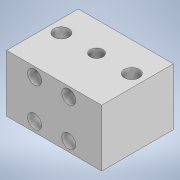
# Autodesk Inventor part: NewSink
Saved by Autodesk Inventor 2020 (Build 240168000, 168)
## iProperties
Created: 2019-09-11
Part Number: NewSink
Material: Generic
Document SubType Name: Modeling
Designer: colman
Density: 1 g/cm^3
Appearance: Default
Author: colman
Autodesk Inventor part; units mm, degrees
ref_plane "YZ Plane" through (0, 0, 0) normal (1, 0, 0) x (0, 1, 0)
ref_plane "XZ Plane" through (0, 0, 0) normal (0, 1, 0) x (-1, 0, 0)
ref_plane "XY Plane" through (0, 0, 0) normal (0, 0, 1) x (1, 0, 0)
sketch "Sketch1" plane through (0, 0, 0) normal (0, 0, 1) x (1, 0, 0)
  line L0 (8.25, 4.95) -> (-8.25, 4.95)
  line L1 (-8.25, 4.95) -> (-8.25, -4.95)
  line L2 (-8.25, -4.95) -> (8.25, -4.95)
  line L3 (8.25, -4.95) -> (8.25, 4.95)
  point P0 (0, 0)
  dimension "d19" = 9.9
  constraints: 8 end point, 2 parallel, 1 horizontal, 1 perpendicular
  measures "d19" distance of L1.end L0.end
extrude "Box" add sketch "Sketch1" along normal mid plane 12.446
sketch "Sketch3" plane through (0, 0, -6.223) normal (0, 0, -1) x (-1, 0, 0)
  line L0 (-5.08, 0) -> (5.08, 0) construction
  line L1 (-4.75, 0) -> (4.75, 0) construction
  line L2 (-2.972, -1.778) -> (2.972, -1.778)
  line L3 (2.972, 1.778) -> (-2.972, 1.778)
  arc A0 (-2.972, 1.778) -> (-2.972, -1.778) centre (-2.972, 0) ccw
  arc A1 (2.972, -1.778) -> (2.972, 1.778) centre (2.972, 0) ccw
  point P0 (0, 0)
  point P1 (0, 0)
  point P2 (0, 0)
  dimension "d31" = 9.5
  constraints: 12 end point, 6 point on circle, 4 point on line, 4 tangent, 2 centre point, 2 midpoint, 1 parallel
  measures "d31" distance of L1.start L1.end
extrude "Slot" cut sketch "Sketch3" against normal blind 10.16
sketch "Sketch4" plane through (0, 0, -6.223) normal (0, 0, -1) x (-1, 0, 0)
  circle A0 centre (-2.5426, 3.364) radius 1.2
  line L0 (-2.972, 1.778) -> (2.972, 1.778) projected
  line L1 (8.25, 4.95) -> (-8.25, 4.95) projected
  point P0 (0, 0)
  dimension "d32" = 2.4
  dimension "d33" = 3.172
  dimension "d34" = 1.586
  constraints: 1 centre point
  measures "d32" diameter of A0
  measures "d33" distance between parallel lines of L0 L1
  measures "d34" distance from line of A0.centre L1
extrude "MountingHole" cut sketch "Sketch4" against normal blind 12.5
pattern_linear "Mounting Holes" count 2 spacing 5.92 along (-1, 0, 0) count 2 spacing 6.648 along (0, -1, 0) of "MountingHole"
sketch "Sketch6" plane through (-8.25, 4.95, 6.223) normal (0, 1, 0) x (1, 0, 0)
  circle A0 centre (8.25, 7.366) radius 1.105
  point P0 (8.25, 6.223)
  dimension "d20" = 2.21
  constraints: 1 centre point
  measures "d20" diameter of A0
extrude "CentralSMAHole" cut sketch "Sketch6" against normal blind 10
sketch "Sketch8" plane through (-8.25, 4.95, 6.223) normal (0, 1, 0) x (1, 0, 0)
  circle A0 centre (14.36, 7.366) radius 1.295
  point P0 (8.25, 6.223)
  dimension "d23" = 2.59
  constraints: 1 centre point
  measures "d23" diameter of A0
extrude "SMAMounting" cut sketch "Sketch8" against normal blind 10
pattern_linear "SMAMountingHoles" count 2 spacing 12.22 along (-1, 0, 0) of "SMAMounting"
equation "\"d34\" = 0.5 * d33"
body "Solid1"
